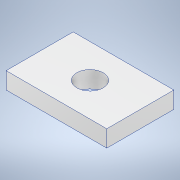
# Autodesk Inventor part: lock ring 1 supp
Saved by Autodesk Inventor 2021 (Build 250183000, 183)
## iProperties
Created: 2021-03-30
Part Number: lock ring 1 supp
Material: Aluminum 6061
Document SubType Name: Modeling
Designer: Work
Density: 2.7 g/cm^3
Appearance: Aluminum - Flat
Mass: 1.90712 g
Surface Area: 6.96208 cm^2
Volume: 0.70634 cm^3
Author: Work
Autodesk Inventor part; units mm, degrees
ref_plane "YZ Plane" through (0, 0, 0) normal (1, 0, 0) x (0, 1, 0)
ref_plane "XZ Plane" through (0, 0, 0) normal (0, 1, 0) x (-1, 0, 0)
ref_plane "XY Plane" through (0, 0, 0) normal (0, 0, 1) x (1, 0, 0)
sketch "Sketch1" plane through (0, 0, 0) normal (0, 1, 0) x (-1, 0, 0)
  line L0 (9.525, 6.35) -> (-9.525, 6.35)
  line L1 (-9.525, 6.35) -> (-9.525, -6.35)
  line L2 (-9.525, -6.35) -> (9.525, -6.35)
  line L3 (9.525, -6.35) -> (9.525, 6.35)
  line L4 (9.525, 6.35) -> (-9.525, -6.35) construction
  line L5 (-9.525, 6.35) -> (9.525, -6.35) construction
  point P0 (0, 0)
  point P1 (0, 0)
  dimension "d1" = 19.05
  dimension "d11" = 12.7
  constraints: 12 end point, 2 midpoint, 2 parallel, 1 coincident, 1 horizontal, 1 perpendicular
  measures "d1" distance of L1.end L2.end
  measures "d11" distance of L2.end L0.start
extrude "Extrusion1" add sketch "Sketch1" along normal blind 3.175
hole "Hole1" at (0, 0, 0) direction (0, 1, 0) diameter 4.9784 end through all clearance for "Flat Head Machine Screw (82)" size "#10" standard "Ansi Unified Screw Threads"
equation "\"height\" = 203.2"
equation "\"thickness\" = 12.7"
equation "\"shaftDiam\" = 6.35"
equation "\"shaftSpace\" = 1.5875"
equation "\"stageSpace\" = 2.54"
equation "\"stageAngle\" = 15deg"
equation "\"bearingDiam\" = 9.5504"
equation "\"FlangeDiam\" = 12.7"
equation "\"FlangeDepth\" = 1.5875"
equation "\"smallFilet\" = 0.39687"
equation "\"ringDiam\" = 96.46608"
equation "\"stockHeight\" = 50.8"
equation "\"stockWidth\" = 76.2"
equation "\"stockRad\" = 9.525"
equation "\"stockGuage\" = 3.175"
equation "\"groundActu\" = 304.8"
equation "\"baseWidth\" = 1066.8"
equation "\"baseDepth\" = 254"
equation "\"capThickness\" = 3.175"
equation "\"sup1Len\" = 660.4"
equation "\"sup1Ang\" = 22.619865deg"
equation "\"sup2Len\" = 2079.37366"
equation "\"sup2Ang\" = 8.959949deg"
equation "\"supVertLen\" = 955.13561"
equation "\"supSideLen\" = 1531.12879"
equation "\"supSideAng\" = 19.376933deg"
body "Solid1"
